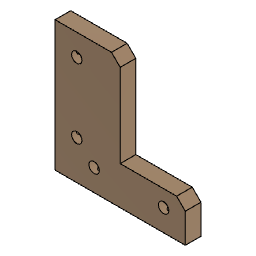
Base Brace L (Autodesk Fusion 360 design; units mm, degrees)
Autodesk Fusion 360 part; units mm, degrees
sketch "Front" plane through (0, 0, 0) normal (0, 1, 0) x (1, 0, 0)
  line L0 (0, 0) -> (150, 0)
  line L1 (150, 0) -> (150, -44)
  line L2 (75, -150) -> (0, -150)
  line L3 (0, -150) -> (0, 0)
  line L4 (75, -150) -> (75, -44)
  line L5 (75, -44) -> (150, -44)
  line L6 (25, -150) -> (25, 0) construction
  line L7 (0, -25) -> (150, -25) construction
  circle A0 centre (45, -25) radius 6
  circle A1 centre (125, -25) radius 6
  circle A2 centre (25, -45) radius 6
  circle A3 centre (25, -125) radius 6
  dimension "d1" = 150
  dimension "d2" = 150
  dimension "d5" = 75
  dimension "d6" = 106
  dimension "d7" = 25
  dimension "d8" = 25
  dimension "d9" = 12
  dimension "d10" = 12
  dimension "d11" = 12
  dimension "d12" = 12
  dimension "d13" = 80
  dimension "d14" = 80
  dimension "d15" = 45
  dimension "d16" = 45
  constraint horizontal L0
  constraint vertical L1
  constraint horizontal L2
  constraint vertical L3
  constraint coincident L0.start L3.end
  constraint vertical L4
  constraint horizontal L5
  constraint coincident L0 L6.end
  constraint perpendicular L0 L6
  constraint coincident L3 L7.start
  constraint coincident L1 L7.end
  constraint perpendicular L1 L7
  constraint coincident L7 A0.centre
  constraint coincident L7 A1.centre
  constraint coincident L6 A2.centre
  constraint coincident L6 A3.centre
  measures "d1" distance of L0.start L0.end
  measures "d2" distance of L0.start L2.end
  measures "d5" distance of L4.end L1.end
  measures "d6" distance of L2.start L4.end
  measures "d7" distance of L0 L7
  measures "d8" distance of L3 L6
  measures "d9" diameter of A0
  measures "d10" diameter of A1
  measures "d11" diameter of A2
  measures "d12" diameter of A3
  measures "d13" distance of A2.centre A3.centre
  measures "d14" distance of A0.centre A1.centre
  measures "d15" distance of L3 A0.centre
  measures "d16" distance of L0 A2.centre
extrude "Extrude1" add sketch "Front" along normal blind 18
chamfer "Chamfer1" distance 10 angle 45 1 edges at (75, 9, 150)
chamfer "Chamfer2" distance 10 angle 45 1 edges at (150, 9, 44)
sketch "Left" plane through (0, 0, 0) normal (-1, 0, 0) x (0, -1, 0)
  line L0 (0, 0) -> (0, 150)
  line L1 (0, 150) -> (-18, 150)
  line L2 (-18, 150) -> (-18, 0)
  line L3 (-18, 0) -> (0, 0)
  line L4 (-9, 0) -> (-9, 150) construction
  circle A0 centre (-9, 45) radius 3.5
  circle A1 centre (-9, 125) radius 3.5
  dimension "d21" = 7
  dimension "d22" = 7
  dimension "d23" = 45
  dimension "d24" = 80
  constraint midpoint L3 L4.start
  constraint midpoint L1 L4.end
  constraint coincident L4 A0.centre
  constraint coincident L4 A1.centre
  measures "d21" diameter of A0
  measures "d22" diameter of A1
  measures "d23" distance of L3 A0.centre
  measures "d24" distance of A0.centre A1.centre
extrude "Extrude2" cut sketch "Left" against normal blind 35 contours A0 | A1
sketch "Bottom" plane through (0, 0, 0) normal (0, 0, -1) x (1, 0, 0)
  line L0 (150, 0) -> (0, 0)
  line L1 (0, 0) -> (0, -18)
  line L2 (0, -18) -> (150, -18)
  line L3 (150, -18) -> (150, 0)
  line L4 (0, -9) -> (150, -9) construction
  circle A0 centre (45, -9) radius 3.5
  circle A1 centre (125, -9) radius 3.5
  dimension "d27" = 7
  dimension "d28" = 7
  dimension "d29" = 45
  dimension "d30" = 80
  constraint midpoint L1 L4.start
  constraint midpoint L3 L4.end
  constraint coincident L4 A0.centre
  constraint coincident L4 A1.centre
  measures "d27" diameter of A0
  measures "d28" diameter of A1
  measures "d29" distance of L1 A0.centre
  measures "d30" distance of A0.centre A1.centre
extrude "Extrude3" cut sketch "Bottom" against normal blind 35 contours A0 | A1
named bodies: "Base Brace L"
